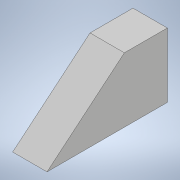
# Autodesk Inventor part: FP Struts
Saved by Autodesk Inventor 2020 (Build 240168000, 168)
## iProperties
Created: 2021-04-23
Part Number: FP Struts
Material: Generic
Document SubType Name: Modeling
Designer: austi
Density: 1 g/cm^3
Appearance: Default
Author: austi
Autodesk Inventor part; units mm, degrees
ref_plane "YZ Plane" through (0, 0, 0) normal (1, 0, 0) x (0, 1, 0)
ref_plane "XZ Plane" through (0, 0, 0) normal (0, 1, 0) x (-1, 0, 0)
ref_plane "XY Plane" through (0, 0, 0) normal (0, 0, 1) x (1, 0, 0)
sketch "Sketch1" plane through (0, 0, 0) normal (0, 1, 0) x (-1, 0, 0)
  line L0 (0, 0) -> (0, -28)
  line L1 (0, 0) -> (15, 0)
  line L2 (15, 0) -> (15, -10)
  line L3 (15, -10) -> (0, -28)
  dimension "d0" = 28
  dimension "d2" = 15
  dimension "d3" = 10
  dimension "d4" = 140.194
  dimension "d5" = 39.806
  constraints: 8 end point, 1 horizontal, 1 perpendicular, 1 vertical
  measures "d0" distance of L0.start L0.end
  measures "d2" distance of L0.start L1.end
  measures "d3" distance of L1.end L2.end
  measures "d4" angle of L3 L2
  measures "d5" angle of L0 L3
extrude "Extrusion1" add sketch "Sketch1" along normal blind 8
body "Solid1"
